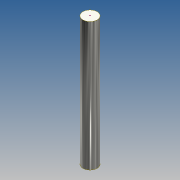
# Autodesk Inventor part: Verin
Saved by Autodesk Inventor 2021.3 (Build 253353000, 353)
## iProperties
Created: 2023-04-12
Part Number: Verin
Material: Steel
Document SubType Name: Modeling
Designer: cedric.clivaz
Density: 7.85 g/cm^3
Appearance: Silver
Author: cedric.clivaz
Autodesk Inventor part; units mm, degrees
ref_plane "YZ Plane" through (0, 0, 0) normal (1, 0, 0) x (0, 1, 0)
ref_plane "XZ Plane" through (0, 0, 0) normal (0, 1, 0) x (-1, 0, 0)
ref_plane "XY Plane" through (0, 0, 0) normal (0, 0, 1) x (1, 0, 0)
sketch "Sketch2" plane through (0, 0, 0) normal (0, 0, 1) x (1, 0, 0)
  circle A0 centre (0, 0) radius 1.5
  dimension "d0" = 3
  constraints: 1 centre point, 1 coincident
  measures "d0" diameter of A0
extrude "Extrusion1" add sketch "Sketch2" along normal blind 27
sketch "Sketch3" plane through (0, 0, 27) normal (0, 0, 1) x (1, 0, 0)
  point P0 (0, 0)
body "Solid1"
